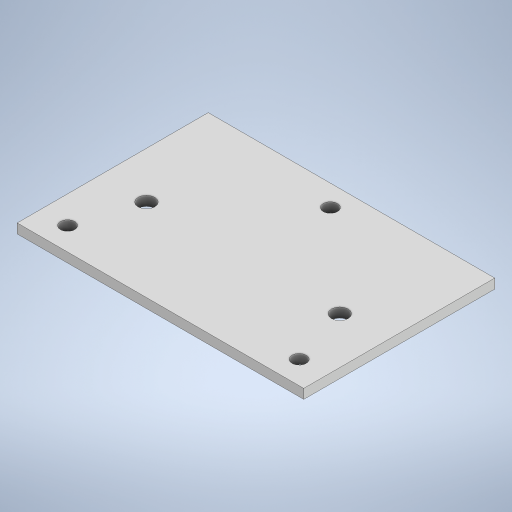
# Autodesk Inventor part: dociazenie
Saved by Autodesk Inventor 2023 (Build 270158000, 158)
## iProperties
Created: 2023-09-02
Part Number: dociazenie
Material: Ogólny
Document SubType Name: Modeling
Designer: Kamil
Density: 1 g/cm^3
Appearance: Domyślna
Author: Kamil
Autodesk Inventor part; units mm, degrees
ref_plane "YZ Plane" through (0, 0, 0) normal (1, 0, 0) x (0, 1, 0)
ref_plane "XZ Plane" through (0, 0, 0) normal (0, 1, 0) x (-1, 0, 0)
ref_plane "XY Plane" through (0, 0, 0) normal (0, 0, 1) x (1, 0, 0)
sketch "Szkic1" plane through (0, 0, 0) normal (0, 1, 0) x (-1, 0, 0)
  line L0 (-75.7688, 32.9192) -> (-75.7688, 6.9192)
  line L1 (-75.7688, 6.9192) -> (-15.7688, 6.9192)
  line L2 (-15.7688, 6.9192) -> (-15.7688, 32.9192)
  circle A0 centre (-70.0174, 42.1278) radius 1.5
  circle A1 centre (-21.5202, 42.1278) radius 1.5
  circle A2 centre (-45.7688, 11.3479) radius 1.5
  circle A3 centre (-25.5188, 29.6192) radius 1.75
  circle A4 centre (-66.0188, 29.6192) radius 1.75
  line L3 (-75.7688, 6.9192) -> (-15.7688, 6.9192)
  line L4 (-15.7688, 6.9192) -> (-15.7688, 46.9192)
  line L5 (-15.7688, 46.9192) -> (-75.7688, 46.9192)
  line L6 (-75.7688, 46.9192) -> (-75.7688, 6.9192)
  point P0 (0, 0)
  dimension "d0" = 40
  constraints: 14 end point, 5 centre point, 2 parallel, 1 horizontal, 1 perpendicular
  measures "d0" distance of L5.start L3.end
extrude "Wyciągnięcie proste1" add sketch "Szkic1" along normal blind 2
